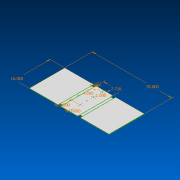
# Autodesk Inventor part: Flat Ramp Using 1__16 Gray Tinted Polycarbonate Sheet (36 x 72) (217-6627)
Saved by Autodesk Inventor 2022 (Build 260153000, 153)
## iProperties
Created: 2022-04-09
Part Number: Flat Ramp Using 1__16 Gray Tinted Polycarbonate Sheet (36 x 72) (217-6627)
Material: Generic
Document SubType Name: Modeling
Designer: score_nygvs6w
Density: 1 g/cm^3
Appearance: Default
Author: score_nygvs6w
Autodesk Inventor part; units mm, degrees
ref_plane "YZ Plane" through (0, 0, 0) normal (1, 0, 0) x (0, 1, 0)
ref_plane "XZ Plane" through (0, 0, 0) normal (0, 1, 0) x (-1, 0, 0)
ref_plane "XY Plane" through (0, 0, 0) normal (0, 0, 1) x (1, 0, 0)
sketch "Sketch1" plane through (0, 0, 0) normal (0, 1, 0) x (-1, 0, 0)
  line L0 (98.1647, -203.2) -> (-98.1647, -203.2)
  line L1 (-98.1647, -203.2) -> (-98.1647, 203.2)
  line L2 (-98.1647, 203.2) -> (98.1647, 203.2)
  line L3 (98.1647, 203.2) -> (98.1647, -203.2)
  line L4 (457.2, -203.2) -> (126.6529, -203.2)
  line L5 (126.6529, -203.2) -> (126.6529, 203.2)
  line L6 (126.6529, 203.2) -> (457.2, 203.2)
  line L7 (457.2, 203.2) -> (457.2, -203.2)
  line L8 (126.6529, -177.8) -> (98.1647, -177.8)
  line L9 (98.1647, -177.8) -> (98.1647, 177.8)
  line L10 (98.1647, 177.8) -> (126.6529, 177.8)
  line L11 (126.6529, 177.8) -> (126.6529, -177.8)
  line L12 (-98.1647, 177.8) -> (-126.6529, 177.8)
  line L13 (-126.6529, 177.8) -> (-126.6529, -177.8)
  line L14 (-126.6529, -177.8) -> (-98.1647, -177.8)
  line L15 (-98.1647, -177.8) -> (-98.1647, 177.8)
  line L16 (-126.6529, -203.2) -> (-457.2, -203.2)
  line L17 (-457.2, -203.2) -> (-457.2, 203.2)
  line L18 (-457.2, 203.2) -> (-126.6529, 203.2)
  line L19 (-126.6529, 203.2) -> (-126.6529, -203.2)
  point P0 (0, 0)
  point P1 (0, -203.2)
  point P2 (98.1647, 0)
  point P3 (98.1647, 0)
  point P4 (0, -76.2)
  point P5 (0, 76.2)
  point P6 (0, -177.8)
  point P7 (0, 177.8)
  dimension "d0" = 25.4
  dimension "d1" = 28.4882
  dimension "d3" = 196.3293
  dimension "d4" = 406.4
  dimension "d5" = 914.4
  dimension "d8" = 101.6
  dimension "d9" = 101.6
  dimension "d10" = 25.4
  dimension "d11" = 25.4
  constraints: 40 end point, 10 parallel, 8 point on line, 5 horizontal, 5 perpendicular, 5 vertical alignment, 4 collinear, 3 midpoint, 1 coincident, 1 horizontal alignment
  measures "d0" distance between parallel lines of L0 L8
  measures "d1" distance between parallel lines of L5 L3
  measures "d3" distance between parallel lines of L1 L3
  measures "d4" distance between parallel lines of L6 L4
  measures "d5" distance between parallel lines of L17 L7
  measures "d8" distance of point (0, -76.2) point (0, -177.8)
  measures "d9" distance of point (0, 177.8) point (0, 76.2)
  measures "d10" distance from line of L0 point (0, -177.8)
  measures "d11" distance from line of L2 point (0, 177.8)
extrude "Extrusion1" add sketch "Sketch1" along normal blind 1.6256
hole "Hole1" at (0, 0, -76.2) at (0, 0, 76.2) at (0, 0, -177.8) at (0, 0, 177.8) direction (0, 1, 0) diameter 4.572 end through all
equation "\"d9\" = d8"
equation "\"d11\" = d10"
body "Solid1"
